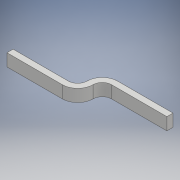
# Autodesk Inventor part: SSSS
Saved by Autodesk Inventor 2018 (Build 220112000, 112)
## iProperties
Created: 2018-02-07
Part Number: SSSS
Material: Generic
Document SubType Name: Modeling
Designer: eroldan
Density: 1 g/cm^3
Appearance: Default
Author: eroldan
Autodesk Inventor part; units mm, degrees
ref_plane "XZ Plane" through (0, 0, 0) normal (0, 1, 0) x (-1, 0, 0)
ref_plane "XY Plane" through (0, 0, 0) normal (0, 0, 1) x (1, 0, 0)
sketch "Sketch2" plane through (0, 0, 0) normal (0, 0, 1) x (1, 0, 0)
  line L0 (-8, 0.1705) -> (10, 0.1705)
  line L1 (36, 8.1705) -> (18, 8.1705)
  line L2 (14, 4.1705) -> (14, 4.1705)
  arc A0 (18, 8.1705) -> (14, 4.1705) centre (18, 4.1705) ccw
  arc A1 (10, 0.1705) -> (14, 4.1705) centre (10, 4.1705) ccw
  point P0 (14, 0.1705)
  point P1 (14, 8.1705)
  dimension "d9" = 44
  dimension "d15" = 8
  dimension "d16" = 22
  dimension "d17" = 22
  dimension "d24" = 4
  constraints: 6 end point, 4 point on circle, 4 point on line, 4 tangent, 2 centre point, 2 horizontal, 1 equal radius, 1 vertical
  measures "d9" horizontal distance of L0.start L1.start
  measures "d15" distance of point (14, 0.171) point (14, 8.171)
  measures "d16" distance of L0.start point (14, 0.171)
  measures "d17" distance of L1.start point (14, 8.171)
  measures "d24" radius of A0
ref_plane "Work Plane1" through (36, 8.1705, 0) normal (1, 0, 0) x (0, 1, 0)
sketch "Sketch3" plane through (36, 8.1705, 0) normal (1, 0, 0) x (0, 1, 0)
  line L0 (-1, 2) -> (-1, -2)
  line L1 (-1, -2) -> (1, -2)
  line L2 (1, -2) -> (1, 2)
  line L3 (1, 2) -> (-1, 2)
  line L4 (-1, 2) -> (1, -2) construction
  line L5 (-1, -2) -> (1, 2) construction
  point P0 (-8.1705, 0)
  point P1 (0, 0)
  dimension "d20" = 4
  dimension "d21" = 2
  constraints: 12 end point, 2 midpoint, 2 parallel, 1 perpendicular, 1 vertical
  measures "d20" distance of L0.start L0.end
  measures "d21" distance of L1.end L0.end
sweep "Sweep1" add profiles "Sketch3" path "Sketch2"
body "Solid2"
